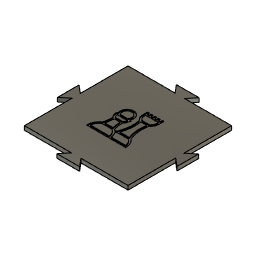
Lab#3.4.1 (Autodesk Fusion 360 design; units mm, degrees)
Autodesk Fusion 360 part; units mm, degrees
sketch "Puzzle" plane through (0, 0, 0) normal (0, 0, 1) x (1, 0, 0)
  line L0 (60.739, 0) -> (89.261, 0)
  line L1 (150, -61.4277) -> (150, -88.5723)
  line L2 (89.261, -150) -> (60.739, -150)
  line L3 (0, -88.5723) -> (0, -61.4277)
  line L4 (60.739, -150) -> (69.0473, -140)
  line L5 (89.261, -150) -> (80.9527, -140)
  line L6 (60.739, 0) -> (69.0473, -10)
  line L7 (89.261, 0) -> (80.9527, -10)
  line L8 (10, -69.8765) -> (0, -61.4277)
  line L9 (10, -80.1235) -> (0, -88.5723)
  line L10 (140, -80.1235) -> (150, -88.5723)
  line L11 (140, -69.8765) -> (150, -61.4277)
  line L12 (10, -140) -> (10, -80.1235)
  line L13 (10, -69.8765) -> (10, -10)
  line L14 (10, -10) -> (69.0473, -10)
  line L15 (80.9527, -10) -> (140, -10)
  line L16 (140, -10) -> (140, -69.8765)
  line L17 (140, -80.1235) -> (140, -140)
  line L18 (140, -140) -> (80.9527, -140)
  line L19 (69.0473, -140) -> (10, -140)
  dimension "d3" = 10
  dimension "d4" = 10
  dimension "d5" = 10
  dimension "d6" = 10
  constraint horizontal L0
  constraint vertical L1
  constraint horizontal L2
  constraint vertical L3
  constraint horizontal L14
  constraint vertical L16
  constraint horizontal L18
  constraint vertical L12
  constraint coincident L4.end L18
  constraint coincident L8.start L12
  constraint collinear L12 L13
  constraint collinear L14 L15
  constraint collinear L16 L17
  constraint collinear L18 L19
  measures "d3" distance of L3 L12
  measures "d4" distance of L1 L16
  measures "d5" distance of L0 L14
  measures "d6" distance of L2 L18
extrude "Extrude1" add sketch "Puzzle" along normal blind 5
sketch "Chess_Pieces" plane through (0, 0, 5) normal (0, 0, 1) x (-1, 0, 0)
  line L0 (-89.261, 150) -> (-80.9527, 140)
  line L1 (-80.9527, 140) -> (-140, 140)
  line L2 (-140, 140) -> (-140, 80.1235)
  line L3 (-140, 80.1235) -> (-150, 88.5723)
  line L4 (-150, 88.5723) -> (-150, 61.4277)
  line L5 (-150, 61.4277) -> (-140, 69.8765)
  line L6 (-140, 69.8765) -> (-140, 10)
  line L7 (-140, 10) -> (-80.9527, 10)
  line L8 (-80.9527, 10) -> (-89.261, 0)
  line L9 (-89.261, 0) -> (-60.739, 0)
  line L10 (-60.739, 0) -> (-69.0473, 10)
  line L11 (-69.0473, 10) -> (-10, 10)
  line L12 (-10, 10) -> (-10, 69.8765)
  line L13 (-10, 69.8765) -> (0, 61.4277)
  line L14 (0, 61.4277) -> (0, 88.5723)
  line L15 (0, 88.5723) -> (-10, 80.1235)
  line L16 (-10, 80.1235) -> (-10, 140)
  line L17 (-10, 140) -> (-69.0473, 140)
  line L18 (-69.0473, 140) -> (-60.739, 150)
  line L19 (-60.739, 150) -> (-89.261, 150)
  spline S0 degree 3 poles (-91.223, 87.4243) (-90.9389, 86.5168) (-90.6193, 85.5352) (-90.2712, 84.5007) knots 0 0 0 0 1 1 1 1
  spline S1 degree 3 poles (-90.2712, 84.5007) (-87.8865, 77.3988) (-87.3842, 69.7773) (-88.8127, 62.428) knots 0 0 0 0 1 1 1 1
  spline S2 degree 3 poles (-88.8127, 62.428) (-91.4249, 60.4902) (-92.97, 57.4402) (-92.97, 54.1742) knots 0 0 0 0 1 1 1 1
  line L20 (-92.97, 54.1742) -> (-92.9642, 47.8864)
  line L21 (-92.9642, 47.8864) -> (-90.6618, 47.8864)
  line L22 (-90.6618, 47.8864) -> (-90.6618, 50.2779)
  line L23 (-90.6618, 50.2779) -> (-88.4095, 50.2779)
  line L24 (-88.4095, 50.2779) -> (-88.4095, 47.8864)
  line L25 (-88.4095, 47.8864) -> (-86.107, 47.8864)
  line L26 (-86.107, 47.8864) -> (-86.107, 50.2779)
  line L27 (-86.107, 50.2779) -> (-83.8549, 50.2779)
  line L28 (-83.8549, 50.2779) -> (-83.8549, 47.8864)
  line L29 (-83.8549, 47.8864) -> (-81.5525, 47.8864)
  line L30 (-81.5525, 47.8864) -> (-81.5525, 50.2779)
  line L31 (-81.5525, 50.2779) -> (-79.3002, 50.2779)
  line L32 (-79.3002, 50.2779) -> (-79.3002, 47.8864)
  line L33 (-79.3002, 47.8864) -> (-76.9978, 47.8864)
  line L34 (-76.9978, 47.8864) -> (-76.9978, 50.2779)
  line L35 (-76.9978, 50.2779) -> (-74.7455, 50.2779)
  line L36 (-74.7455, 50.2779) -> (-74.7455, 47.8864)
  line L37 (-74.7455, 47.8864) -> (-72.4431, 47.8864)
  line L38 (-72.4431, 47.8864) -> (-72.4254, 54.1743)
  spline S3 degree 3 poles (-72.4254, 54.1743) (-72.4254, 57.4402) (-73.9705, 60.4902) (-76.5826, 62.4282) knots 0 0 0 0 1 1 1 1
  spline S4 degree 3 poles (-76.5826, 62.4282) (-78.0114, 69.7787) (-77.5086, 77.4001) (-75.122, 84.5018) knots 0 0 0 0 1 1 1 1
  spline S5 degree 3 poles (-75.122, 84.5018) (-74.7694, 85.5551) (-74.4504, 86.5361) (-74.1724, 87.4243) knots 0 0 0 0 1 1 1 1
  spline S6 degree 3 poles (-74.1724, 87.4243) (-73.5906, 87.8508) (-73.0414, 88.3206) (-72.5295, 88.8289) knots 0 0 0 0 1 1 1 1
  spline S7 degree 3 poles (-72.5295, 88.8289) (-71.8237, 88.1393) (-71.0436, 87.518) (-70.1949, 86.9815) knots 0 0 0 0 1 1 1 1
  spline S8 degree 3 poles (-70.1949, 86.9815) (-69.3275, 83.598) (-68.8115, 80.129) (-68.6574, 76.6506) knots 0 0 0 0 1 1 1 1
  spline S9 degree 2 poles (-68.6574, 76.6506) (-68.6444, 76.3592) (-68.6196, 75.527) knots 0 0 0 1 1 1
  spline S10 degree 3 poles (-68.6196, 75.527) (-70.5678, 73.8023) (-71.6739, 71.3596) (-71.6739, 68.7373) knots 0 0 0 0 1 1 1 1
  line L39 (-71.6739, 68.7373) -> (-71.6739, 67.5861)
  line L40 (-71.6739, 67.5861) -> (-70.0307, 67.5861)
  spline S11 degree 3 poles (-70.0307, 67.5861) (-70.6401, 66.4066) (-70.9658, 65.0887) (-70.9658, 63.7437) knots 0 0 0 0 1 1 1 1
  spline S12 degree 3 poles (-70.9658, 63.7437) (-70.9658, 59.1281) (-67.2107, 55.373) (-62.5951, 55.373) knots 0 0 0 0 1 1 1 1
  spline S13 degree 3 poles (-62.5951, 55.373) (-57.9793, 55.373) (-54.2242, 59.1281) (-54.2242, 63.7437) knots 0 0 0 0 1 1 1 1
  spline S14 degree 3 poles (-54.2242, 63.7437) (-54.2242, 65.0887) (-54.5499, 66.4068) (-55.1593, 67.5861) knots 0 0 0 0 1 1 1 1
  line L41 (-55.1593, 67.5861) -> (-53.5161, 67.5861)
  line L42 (-53.5161, 67.5861) -> (-53.5161, 68.7373)
  spline S15 degree 3 poles (-53.5161, 68.7373) (-53.5161, 71.3722) (-54.6305, 73.8225) (-56.5938, 75.5481) knots 0 0 0 0 1 1 1 1
  spline S16 degree 3 poles (-56.5938, 75.5481) (-56.5091, 79.3901) (-55.9829, 83.2265) (-55.0288, 86.9601) knots 0 0 0 0 1 1 1 1
  spline S17 degree 3 poles (-55.0288, 86.9601) (-50.8946, 89.5567) (-48.3461, 94.1389) (-48.3461, 99.0357) knots 0 0 0 0 1 1 1 1
  line L43 (-48.3461, 99.0357) -> (-48.3461, 100.2048)
  line L44 (-48.3461, 100.2048) -> (-97.1323, 100.2048)
  line L45 (-97.1323, 100.2048) -> (-97.1323, 99.0715)
  spline S18 degree 3 poles (-97.1323, 99.0715) (-97.1323, 94.4677) (-94.9306, 90.1438) (-91.223, 87.4243) knots 0 0 0 0 1 1 1 1
  line L46 (-74.728, 54.1743) -> (-74.728, 52.5804)
  line L47 (-74.728, 52.5804) -> (-90.6678, 52.5804)
  line L48 (-90.6678, 52.5804) -> (-90.6678, 54.1743)
  spline S19 degree 3 poles (-90.6678, 54.1743) (-90.6678, 56.7217) (-89.453, 59.0978) (-87.4056, 60.6009) knots 0 0 0 0 1 1 1 1
  line L49 (-87.4056, 60.6009) -> (-77.9903, 60.6009)
  spline S20 degree 3 poles (-77.9903, 60.6009) (-75.9428, 59.0978) (-74.728, 56.7217) (-74.728, 54.1743) knots 0 0 0 0 1 1 1 1
  line L50 (-79.0103, 62.9033) -> (-86.3855, 62.9033)
  spline S21 degree 3 poles (-86.3855, 62.9033) (-85.0938, 70.3589) (-85.6761, 78.0492) (-88.0891, 85.2343) knots 0 0 0 0 1 1 1 1
  spline S22 degree 3 poles (-88.0891, 85.2343) (-88.2924, 85.839) (-88.4853, 86.4234) (-88.6672, 86.9863) knots 0 0 0 0 1 1 1 1
  line L51 (-88.6672, 86.9863) -> (-76.7284, 86.9863)
  spline S23 degree 3 poles (-76.7284, 86.9863) (-76.9082, 86.4296) (-77.1009, 85.8445) (-77.3053, 85.234) knots 0 0 0 0 1 1 1 1
  spline S24 degree 3 poles (-77.3053, 85.234) (-79.7189, 78.0504) (-80.3019, 70.3602) (-79.0103, 62.9033) knots 0 0 0 0 1 1 1 1
  line L52 (-58.8799, 76.166) -> (-66.3362, 76.166)
  spline S25 degree 3 poles (-66.3362, 76.166) (-66.4516, 79.6568) (-66.9151, 83.142) (-67.7187, 86.5517) knots 0 0 0 0 1 1 1 1
  line L53 (-67.7187, 86.5517) -> (-57.4995, 86.5517)
  spline S26 degree 3 poles (-57.4995, 86.5517) (-58.302, 83.1423) (-58.7651, 79.6584) (-58.8799, 76.166) knots 0 0 0 0 1 1 1 1
  spline S27 degree 3 poles (-56.527, 63.7436) (-56.527, 60.3974) (-59.2493, 57.6753) (-62.5955, 57.6753) knots 0 0 0 0 1 1 1 1
  spline S28 degree 3 poles (-62.5955, 57.6753) (-65.9416, 57.6753) (-68.6637, 60.3974) (-68.6637, 63.7436) knots 0 0 0 0 1 1 1 1
  spline S29 degree 3 poles (-68.6637, 63.7436) (-68.6637, 65.1455) (-68.1756, 66.5065) (-67.2894, 67.5859) knots 0 0 0 0 1 1 1 1
  line L54 (-67.2894, 67.5859) -> (-57.9013, 67.5859)
  spline S30 degree 3 poles (-57.9013, 67.5859) (-57.0151, 66.5065) (-56.527, 65.1455) (-56.527, 63.7436) knots 0 0 0 0 1 1 1 1
  line L55 (-55.9158, 69.8885) -> (-69.2748, 69.8885)
  spline S31 degree 3 poles (-69.2748, 69.8885) (-69.0125, 71.4287) (-68.2259, 72.8262) (-67.0232, 73.8636) knots 0 0 0 0 1 1 1 1
  line L56 (-67.0232, 73.8636) -> (-58.1677, 73.8636)
  spline S32 degree 3 poles (-58.1677, 73.8636) (-56.9646, 72.8261) (-56.1779, 71.4294) (-55.9158, 69.8885) knots 0 0 0 0 1 1 1 1
  line L57 (-56.3447, 88.8541) -> (-68.8449, 88.8541)
  spline S33 degree 3 poles (-68.8449, 88.8541) (-72.0368, 90.8186) (-74.124, 94.1881) (-74.4859, 97.8845) knots 0 0 0 0 1 1 1 1
  line L58 (-74.4859, 97.8845) -> (-50.7047, 97.8845)
  spline S34 degree 3 poles (-50.7047, 97.8845) (-51.0662, 94.1863) (-53.1523, 90.8191) (-56.3447, 88.8541) knots 0 0 0 0 1 1 1 1
  spline S35 degree 3 poles (-76.7985, 97.9203) (-76.5858, 95.2412) (-75.6142, 92.6961) (-74.0463, 90.5705) knots 0 0 0 0 1 1 1 1
  spline S36 degree 3 poles (-74.0463, 90.5705) (-74.5043, 90.1043) (-74.9984, 89.6752) (-75.5248, 89.2885) knots 0 0 0 0 1 1 1 1
  line L59 (-75.5248, 89.2885) -> (-89.8639, 89.2885)
  spline S37 degree 3 poles (-89.8639, 89.2885) (-92.6666, 91.3467) (-94.4477, 94.4918) (-94.775, 97.9201) knots 0 0 0 0 1 1 1 1
  line L60 (-94.775, 97.9201) -> (-76.7985, 97.9201)
  line L61 (-76.7985, 97.9201) -> (-76.7985, 97.9203)
extrude "Extrude2" cut sketch "Chess_Pieces" against normal blind 1 contours S0 S1 S2 L20 L21 L22 L23 L24 L25 L26 L27 L28 L29 L30 L31 L32 L33 L34 L35 L36 L37 L38 S3 S4 S5 S6 S7 S8 S9 S10 L39 L40 S11 S12 S13 S14 L41 L42 S15 S16 S17 L43 L44 L45 S18
named bodies: "Lab#3.4.1"
